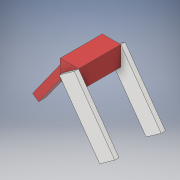
# Autodesk Inventor part: structure
Saved by Autodesk Inventor 2019 (Build 230136000, 136)
## iProperties
Created: 2020-05-27
Part Number: structure
Material: Genérico
Document SubType Name: Modeling
Designer: alejo
Density: 1 g/cm^3
Appearance: Valor por defecto
Author: alejo
Autodesk Inventor part; units mm, degrees
ref_plane "YZ Plane" through (0, 0, 0) normal (1, 0, 0) x (0, 1, 0)
ref_plane "XZ Plane" through (0, 0, 0) normal (0, 1, 0) x (-1, 0, 0)
ref_plane "XY Plane" through (0, 0, 0) normal (0, 0, 1) x (1, 0, 0)
sketch "Boceto1" plane through (0, 0, 0) normal (0, 1, 0) x (-1, 0, 0)
  line L0 (15, 34.35) -> (15, -34.35)
  line L1 (15, -34.35) -> (-15, -34.35)
  line L2 (-15, -34.35) -> (-15, 34.35)
  line L3 (-15, 34.35) -> (15, 34.35)
  line L4 (15, 34.35) -> (-15, -34.35) construction
  line L5 (15, -34.35) -> (-15, 34.35) construction
  point P0 (0, 0)
  dimension "d0" = 68.7
  dimension "d1" = 30
  constraints: 12 end point, 2 midpoint, 2 parallel, 1 perpendicular, 1 vertical
  measures "d0" distance of L0.start L0.end
  measures "d1" distance of L0.end L1.end
extrude "Extrusión1" add sketch "Boceto1" along normal blind 32
sketch "Boceto2" plane through (-15, 0, 34.35) normal (0, 0, 1) x (1, 0, 0)
  line L0 (0, 32) -> (30, 32) projected
  line L1 (30, 32) -> (95.8937, -60.4136)
  line L2 (30, 32) -> (143.5, 32) construction
  line L3 (95.8937, -60.4136) -> (71.4672, -77.8304)
  line L4 (71.4672, -77.8304) -> (5.5735, 14.5832)
  line L5 (5.5735, 14.5832) -> (30, 32)
  point P0 (15, 0)
  dimension "d4" = 113.5
  dimension "d5" = 54.51
  dimension "d6" = 30
  dimension "d7" = 90
  constraints: 10 end point, 3 perpendicular, 1 equal length, 1 horizontal
  measures "d4" distance of L0.end L1.end
  measures "d5" angle of L1 L2
  measures "d6" distance of L1.end L3.end
  measures "d7" angle of L1 L3
extrude "Extrusión2" add sketch "Boceto2" along normal blind 7
sketch "Boceto3" plane through (15, 0, -34.35) normal (0, 0, -1) x (-1, 0, 0)
  line L0 (0, 32) -> (-65.8937, -60.4136) projected
  line L1 (-41.4672, -77.8304) -> (14.0283, 0) projected
  line L2 (-65.8937, -60.4136) -> (-41.4672, -77.8304) projected
  line L3 (0, 32) -> (24.4265, 14.5832) projected
  line L4 (0, 32) -> (-65.8937, -60.4136)
  line L5 (-41.4672, -77.8304) -> (-65.8937, -60.4136)
  line L6 (-41.4672, -77.8304) -> (24.4265, 14.5832)
  line L7 (24.4265, 14.5832) -> (0, 32)
  point P0 (15, 0)
  constraints: 8 end point, 3 collinear, 1 perpendicular
extrude "Extrusión3" add sketch "Boceto3" along normal blind 7
sketch "Boceto4" plane through (0, 0, 0) normal (0, 0, 1) x (1, 0, 0)
  line L0 (15, 32) -> (-15, 32) projected
  line L1 (-15, 32) -> (-82.3451, -62.4492)
  line L2 (-15, 32) -> (101, 32) construction
  line L3 (-82.3451, -62.4492) -> (-72.5745, -69.4159)
  line L4 (-72.5745, -69.4159) -> (-15, 11.3303)
  line L5 (-15, 0) -> (-15, 32) projected
  line L6 (-15, 11.3303) -> (-15, 32)
  point P0 (0, 0)
  dimension "d12" = 116
  dimension "d13" = 125.49
  dimension "d14" = 12
  constraints: 10 end point, 2 perpendicular, 1 collinear, 1 equal length, 1 horizontal
  measures "d12" distance of L0.end L1.end
  measures "d13" angle of L1 L2
  measures "d14" distance of L1.end L3.end
extrude "Extrusión4" add sketch "Boceto4" along normal blind 12
